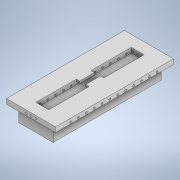
# Autodesk Inventor part: dhillg25_P2_Milestone3
Saved by Autodesk Inventor 2021 (Build 250183000, 183)
## iProperties
Created: 2020-11-14
Part Number: dhillg25_P2_Milestone3
Material: Generic
Document SubType Name: Modeling
Designer: gurle
Density: 1 g/cm^3
Appearance: Default
Author: gurle
Autodesk Inventor part; units mm, degrees
ref_plane "XZ Plane" through (0, 0, 0) normal (0, 1, 0) x (-1, 0, 0)
ref_plane "Work Plane1" through (25, 0, 0) normal (1, 0, 0) x (0, 1, 0)
ref_plane "Work Plane2" through (0, 0, 60) normal (0, 0, 1) x (1, 0, 0)
sketch "Sketch1" plane through (0, 0, 0) normal (0, 1, 0) x (-1, 0, 0)
  line L0 (0, 0) -> (-50, 0)
  line L1 (-50, 0) -> (-50, 120)
  line L2 (-50, 120) -> (0, 120)
  line L3 (0, 120) -> (0, 0)
  line L4 (-18.5, 108.5) -> (-31.5, 108.5)
  line L5 (-31.5, 108.5) -> (-31.5, 11.5)
  line L6 (-31.5, 11.5) -> (-18.5, 11.5)
  line L7 (-18.5, 11.5) -> (-18.5, 108.5)
  dimension "d0" = 50
  dimension "d1" = 120
  dimension "d2" = 13
  dimension "d3" = 97
  dimension "d4" = 11.5
  dimension "d5" = 18.5
  constraints: 16 end point, 4 parallel, 2 horizontal, 2 perpendicular
  measures "d0" distance of L1.end L2.end
  measures "d1" distance of L0.end L1.end
  measures "d2" distance of L6.end L5.end
  measures "d3" distance of L5.end L4.end
  measures "d4" distance between parallel lines of L2 L4
  measures "d5" distance between parallel lines of L3 L7
extrude "Extrusion1" add sketch "Sketch1" along normal blind 3
sketch "Sketch2" plane through (0, 0, 0) normal (0, -1, 0) x (1, 0, 0)
  line L0 (42.5, 115) -> (7.5, 115)
  line L1 (7.5, 115) -> (7.5, 5)
  line L2 (7.5, 5) -> (42.5, 5)
  line L3 (42.5, 5) -> (42.5, 115)
  line L4 (50, 0) -> (0, 0) projected
  line L5 (50, 120) -> (50, 0) projected
  line L6 (0, 0) -> (0, 120) projected
  line L7 (0, 120) -> (50, 120) projected
  dimension "d8" = 35
  dimension "d9" = 110
  dimension "d14" = 7.5
  dimension "d15" = 5
  constraints: 8 end point, 2 parallel, 1 horizontal, 1 perpendicular
  measures "d8" distance of L1.end L2.end
  measures "d9" distance of L2.end L0.start
  measures "d14" distance between parallel lines of L6 L1
  measures "d15" distance between parallel lines of L7 L0
extrude "Extrusion2" add sketch "Sketch2" along normal blind 15 contours L3 L2 L1 L0
sketch "Sketch4" plane through (0, 3, 0) normal (0, 1, 0) x (1, 0, 0)
  line L0 (0, -120) -> (50, -120) projected
  line L1 (0, -120) -> (50, -120)
  line L2 (50, -120) -> (50, 0)
  line L3 (50, 0) -> (0, 0)
  line L4 (0, 0) -> (0, -120)
  line L5 (18.5, -11.5) -> (31.5, -11.5) projected
  line L6 (18.5, -108.5) -> (31.5, -108.5)
  line L7 (31.5, -11.5) -> (18.5, -11.5)
  line L8 (18.5, -108.5) -> (18.5, -11.5) projected
  line L9 (18.5, -67.5) -> (22, -67.5)
  line L10 (22, -67.5) -> (22, -52.5)
  line L11 (22, -52.5) -> (18.5, -52.5)
  line L12 (18.5, -52.5) -> (18.5, -67.5)
  line L13 (31.5, -11.5) -> (31.5, -108.5) projected
  line L14 (31.5, -67.5) -> (28, -67.5)
  line L15 (28, -67.5) -> (28, -52.5)
  line L16 (28, -52.5) -> (31.5, -52.5)
  line L17 (31.5, -52.5) -> (31.5, -67.5)
  line L18 (18.5, -67.5) -> (18.5, -108.5)
  line L19 (31.5, -67.5) -> (31.5, -108.5)
  line L20 (31.5, -52.5) -> (31.5, -11.5)
  line L21 (18.5, -52.5) -> (18.5, -11.5)
  point P0 (0, 0)
  dimension "d16" = 15
  dimension "d17" = 3.5
  dimension "d18" = 3.5
  dimension "d19" = 41
  constraints: 36 end point, 7 parallel, 4 horizontal, 4 point on line, 3 collinear, 3 perpendicular
  measures "d16" distance of L9.end L10.end
  measures "d17" distance of L15.end L16.end
  measures "d18" distance of L10.end L11.end
  measures "d19" distance between parallel lines of L5 L16
extrude "Extrusion3" add sketch "Sketch4" along normal blind 2 contours L4 L3 L2 L0 | L11 L10 L9 L8 | L13 L14 L15 L16
sketch "Sketch6" plane through (18.5, 0, 108.5) normal (1, 0, 0) x (0, 0, -1)
  point P0 (108.5, 0)
  point P1 (3.711, 1.7158)
hole "Hole1" at (18.5, 1.7158, 104.789) direction (-1, 0, 0) diameter 2 end through all
pattern_linear "Rectangular Pattern1" count 12 spacing 8 along (0, 0, -1) of "Hole1"
mirror "Mirror1" about plane through (25, 0, 0) normal (1, 0, 0) of "Hole1", "Rectangular Pattern1"
sketch "Sketch8" plane through (31.5, 0, 108.5) normal (0, 0, -1) x (-1, 0, 0)
  point P0 (31.5, 0)
  point P1 (11.368, 2.2274)
hole "Hole2" at (20.132, 2.2274, 108.5) direction (0, 0, 1) diameter 2 end through all
pattern_linear "Rectangular Pattern2" count 3 spacing 5 along (1, 0, 0) of "Hole2"
mirror "Mirror2" about plane through (0, 0, 60) normal (0, 0, 1) of "Hole2", "Rectangular Pattern2"
body "Solid1"
